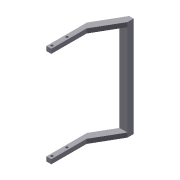
# Autodesk Inventor part: Alça
Saved by Autodesk Inventor 2011 (Build 150239000, 239)
## iProperties
Created: 2010-11-28
Part Number: Alça
Document SubType Name: Modeling
Designer: Milton
Density: 2.71 g/cm^3
Mass: 27.78 g
Surface Area: 68.7628 cm^2
Volume: 10.2509 cm^3
Material: Aluminum-6061
Author: Milton
Autodesk Inventor part; units mm, degrees
ref_plane "YZ Plane" through (0, 0, 0) normal (1, 0, 0) x (0, 1, 0)
ref_plane "XZ Plane" through (0, 0, 0) normal (0, 1, 0) x (-1, 0, 0)
sketch "Sketch1" plane through (0, 0, 0) normal (0, 0, 1) x (1, 0, 0)
  arc A0 (12.2, 9) -> (9.2, 12) centre (9.2, 9) ccw projected
  line L0 (12.7, 12) -> (9.2, 12) projected
  line L1 (12.7, 12) -> (17.8, 6) projected
  line L2 (17.8, 6) -> (17.8, -32.6) projected
  line L3 (17.8, -32.6) -> (12.7, -38.6) projected
  line L4 (12.7, -38.6) -> (-12.7, -38.6) projected
  line L5 (-12.7, -38.6) -> (-17.8, -32.6) projected
  line L6 (-17.8, -32.6) -> (-17.8, 6) projected
  line L7 (-17.8, 6) -> (-12.7, 12) projected
  line L8 (-9.2, 12) -> (-12.7, 12) projected
  arc A1 (-9.2, 12) -> (-12.2, 9) centre (-9.2, 9) ccw projected
  line L9 (-12.2, -30) -> (-12.2, 9) projected
  arc A2 (-12.2, -30) -> (-9.2, -33) centre (-9.2, -30) ccw projected
  line L10 (9.2, -33) -> (-9.2, -33) projected
  arc A3 (9.2, -33) -> (12.2, -30) centre (9.2, -30) ccw projected
  line L11 (12.2, 9) -> (12.2, -30) projected
  circle A4 centre (-15, -29.5) radius 1.35 projected
  circle A5 centre (15, -29.5) radius 1.35 projected
  circle A6 centre (-8.5, -35.8) radius 1.35 projected
  circle A7 centre (-15, -12.5) radius 1.35 projected
  circle A8 centre (-15, 4.5) radius 1.35 projected
  circle A9 centre (8.5, -35.8) radius 1.35 projected
  circle A10 centre (15, -12.5) radius 1.35 projected
  circle A11 centre (15, 4.5) radius 1.35 projected
  line L12 (12.2, -16) -> (12.2, 29.9608)
  line L13 (29.7534, 60.3642) -> (34.7534, 60.3642)
  line L14 (34.7534, 60.3642) -> (34.7534, 53.3642)
  line L15 (34.7534, 53.3642) -> (17.8, 24)
  line L16 (17.8, 24) -> (17.8, -16)
  line L17 (12.2, -16) -> (17.8, -16)
  circle A12 centre (15, -12.5) radius 1.35
  circle A13 centre (15, 4.5) radius 1.35
  line L18 (12.2, 29.9608) -> (29.7534, 60.3642)
  point P0 (0, 0)
  dimension "d1" = 2.7
  dimension "d2" = 2.7
  dimension "d3" = 5.6
  dimension "d4" = 3.5
  dimension "d5" = 40
  dimension "d6" = 30
  dimension "d7" = 7
  dimension "d9" = 5
  constraints: 14 end point, 3 perpendicular, 2 centre point, 2 coincident, 2 point on line, 1 collinear, 1 parallel
  measures "d1" diameter of A12
  measures "d2" diameter of A13
  measures "d3" distance of L12.start L16.end
  measures "d4" distance from line of L17 A10.centre
  measures "d5" distance of L15.end L16.end
  measures "d6" angle of L15 L16
  measures "d7" distance of L13.end L14.end
  measures "d9" distance of L13.start L13.end
extrude "Extrusion1" add sketch "Sketch1" along normal blind 5 contours L12 L0 L1 L2 L17 L11 | L12 L18 L13 L14 L15 L16 L1 L0
sketch "Sketch2" plane through (0, 0, 5) normal (0, 0, 1) x (1, 0, 0)
  line L0 (34.7534, 60.3642) -> (34.7534, 53.3642) projected
  line L1 (29.7534, 60.3642) -> (34.7534, 60.3642) projected
  line L2 (34.7534, 60.3642) -> (29.7534, 60.3642)
  line L3 (34.7534, 60.3642) -> (29.7534, 60.3642) projected
  line L4 (29.7534, 60.3642) -> (25.712, 53.3642)
  line L5 (29.7534, 60.3642) -> (12.2, 29.9608) projected
  line L6 (34.7534, 53.3642) -> (25.712, 53.3642)
  line L7 (34.7534, 53.3642) -> (34.7534, 60.3642)
  point P0 (0, 0)
  constraints: 8 end point, 1 collinear, 1 parallel, 1 perpendicular
ref_plane "Work Plane1" through (12.1861, 4.5831, 113.4) normal (0, 0, -1) x (0, 1, 0)
extrude "Extrusion2" add sketch "Sketch2" along normal up to surface (108.4 mm away)
sketch "Sketch3" plane through (25.712, 53.3642, 113.4) normal (0, 0, 1) x (1, 0, 0)
  line L0 (9.0415, 7) -> (4.0415, 7) projected
  line L1 (4.0415, 7) -> (0, 0) projected
  line L2 (0, 0) -> (9.0415, 0) projected
  line L3 (9.0415, 0) -> (9.0415, 7) projected
  circle A0 centre (-10.712, -48.8642) radius 1.35 projected
  circle A1 centre (-10.712, -65.8642) radius 1.35 projected
  line L4 (-13.512, -23.4034) -> (-13.512, -69.3642) projected
  line L5 (4.0415, 7) -> (-13.512, -23.4034) projected
  line L6 (9.0415, 7) -> (4.0415, 7) projected
  line L7 (9.0415, 0) -> (9.0415, 7) projected
  line L8 (-7.912, -29.3642) -> (9.0415, 0) projected
  line L9 (-7.912, -69.3642) -> (-7.912, -29.3642) projected
  line L10 (-13.512, -69.3642) -> (-7.912, -69.3642) projected
  point P0 (-25.712, -53.3642)
extrude "Extrusion3" add sketch "Sketch3" against normal blind 5 contours L8 L9 L10 L4 L5 L2
body "Solid1"
